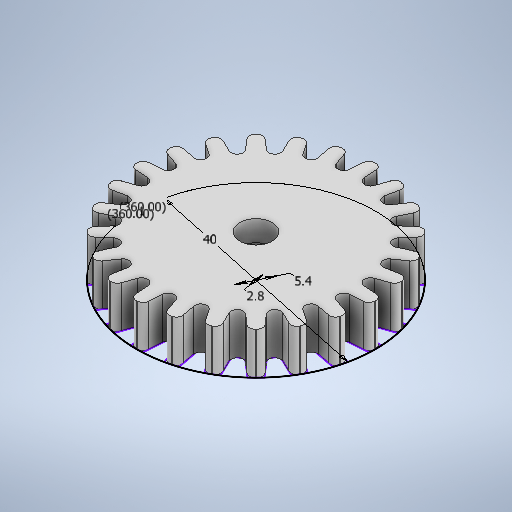
# Autodesk Inventor part: Direcccion3
Saved by Autodesk Inventor 2025.2 (Build 292293000, 293)
## iProperties
Created: 2025-03-19
Part Number: Direcccion3
Material: Genérico
Document SubType Name: Modeling
Designer: angel.dasilva
Density: 1 g/cm^3
Appearance: Valor por defecto
Author: angel.dasilva
Autodesk Inventor part; units mm, degrees
ref_plane "YZ Plane" through (0, 0, 0) normal (1, 0, 0) x (0, 1, 0)
ref_plane "XZ Plane" through (0, 0, 0) normal (0, 1, 0) x (-1, 0, 0)
ref_plane "XY Plane" through (0, 0, 0) normal (0, 0, 1) x (1, 0, 0)
sketch "Boceto1" plane through (0, 0, 0) normal (0, 1, 0) x (-1, 0, 0)
  circle A0 centre (0, 0) radius 20
  line L0 (20, 0) -> (19.975, -0.9997)
  line L1 (19.975, -0.9997) -> (15.9472, -1.2989)
  line L2 (20, 0) -> (19.975, 0.9997)
  line L3 (19.975, 0.9997) -> (15.9472, 1.2989)
  circle A1 centre (0, 0) radius 2.7
  circle A2 centre (0, 0) radius 1.4
  line L4 (19.0356, 6.1355) -> (15.0676, 5.3821)
  line L5 (19.5531, 4.2043) -> (15.74, 2.8728)
  line L6 (16.799, 10.8533) -> (13.1612, 9.0985)
  line L7 (17.7987, 9.1217) -> (14.4601, 6.8487)
  line L8 (13.4176, 14.8313) -> (10.3579, 12.1948)
  line L9 (14.8313, 13.4176) -> (12.1948, 10.3579)
  line L10 (9.1217, 17.7987) -> (6.8487, 14.4601)
  line L11 (10.8533, 16.799) -> (9.0985, 13.1612)
  line L12 (4.2043, 19.5531) -> (2.8728, 15.74)
  line L13 (6.1355, 19.0356) -> (5.3821, 15.0676)
  line L14 (-0.9997, 19.975) -> (-1.2989, 15.9472)
  line L15 (0.9997, 19.975) -> (1.2989, 15.9472)
  line L16 (-6.1355, 19.0356) -> (-5.3821, 15.0676)
  line L17 (-4.2043, 19.5531) -> (-2.8728, 15.74)
  line L18 (-10.8533, 16.799) -> (-9.0985, 13.1612)
  line L19 (-9.1217, 17.7987) -> (-6.8487, 14.4601)
  line L20 (-14.8313, 13.4176) -> (-12.1948, 10.3579)
  line L21 (-13.4176, 14.8313) -> (-10.3579, 12.1948)
  line L22 (-17.7987, 9.1217) -> (-14.4601, 6.8487)
  line L23 (-16.799, 10.8533) -> (-13.1612, 9.0985)
  line L24 (-19.5531, 4.2043) -> (-15.74, 2.8728)
  line L25 (-19.0356, 6.1355) -> (-15.0676, 5.3821)
  line L26 (-19.975, -0.9997) -> (-15.9472, -1.2989)
  line L27 (-19.975, 0.9997) -> (-15.9472, 1.2989)
  line L28 (-19.0356, -6.1355) -> (-15.0676, -5.3821)
  line L29 (-19.5531, -4.2043) -> (-15.74, -2.8728)
  line L30 (-16.799, -10.8533) -> (-13.1612, -9.0985)
  line L31 (-17.7987, -9.1217) -> (-14.4601, -6.8487)
  line L32 (-13.4176, -14.8313) -> (-10.3579, -12.1948)
  line L33 (-14.8313, -13.4176) -> (-12.1948, -10.3579)
  line L34 (-9.1217, -17.7987) -> (-6.8487, -14.4601)
  line L35 (-10.8533, -16.799) -> (-9.0985, -13.1612)
  line L36 (-4.2043, -19.5531) -> (-2.8728, -15.74)
  line L37 (-6.1355, -19.0356) -> (-5.3821, -15.0676)
  line L38 (0.9997, -19.975) -> (1.2989, -15.9472)
  line L39 (-0.9997, -19.975) -> (-1.2989, -15.9472)
  line L40 (6.1355, -19.0356) -> (5.3821, -15.0676)
  line L41 (4.2043, -19.5531) -> (2.8728, -15.74)
  line L42 (10.8533, -16.799) -> (9.0985, -13.1612)
  line L43 (9.1217, -17.7987) -> (6.8487, -14.4601)
  line L44 (14.8313, -13.4176) -> (12.1948, -10.3579)
  line L45 (13.4176, -14.8313) -> (10.3579, -12.1948)
  line L46 (17.7987, -9.1217) -> (14.4601, -6.8487)
  line L47 (16.799, -10.8533) -> (13.1612, -9.0985)
  line L48 (19.5531, -4.2043) -> (15.74, -2.8728)
  line L49 (19.0356, -6.1355) -> (15.0676, -5.3821)
  line L50 (19.975, -0.9997) -> (19.975, 0.9997)
  line L51 (19.5531, 4.2043) -> (19.0356, 6.1355)
  line L52 (17.7987, 9.1217) -> (16.799, 10.8533)
  line L53 (14.8313, 13.4176) -> (13.4176, 14.8313)
  line L54 (10.8533, 16.799) -> (9.1217, 17.7987)
  line L55 (6.1355, 19.0356) -> (4.2043, 19.5531)
  line L56 (0.9997, 19.975) -> (-0.9997, 19.975)
  line L57 (-4.2043, 19.5531) -> (-6.1355, 19.0356)
  line L58 (-9.1217, 17.7987) -> (-10.8533, 16.799)
  line L59 (-13.4176, 14.8313) -> (-14.8313, 13.4176)
  line L60 (-16.799, 10.8533) -> (-17.7987, 9.1217)
  line L61 (-19.0356, 6.1355) -> (-19.5531, 4.2043)
  line L62 (-19.975, 0.9997) -> (-19.975, -0.9997)
  line L63 (-19.5531, -4.2043) -> (-19.0356, -6.1355)
  line L64 (-17.7987, -9.1217) -> (-16.799, -10.8533)
  line L65 (-14.8313, -13.4176) -> (-13.4176, -14.8313)
  line L66 (-10.8533, -16.799) -> (-9.1217, -17.7987)
  line L67 (-6.1355, -19.0356) -> (-4.2043, -19.5531)
  line L68 (-0.9997, -19.975) -> (0.9997, -19.975)
  line L69 (4.2043, -19.5531) -> (6.1355, -19.0356)
  line L70 (9.1217, -17.7987) -> (10.8533, -16.799)
  line L71 (13.4176, -14.8313) -> (14.8313, -13.4176)
  line L72 (16.799, -10.8533) -> (17.7987, -9.1217)
  line L73 (19.0356, -6.1355) -> (19.5531, -4.2043)
  arc A3 (12.1948, -10.3579) -> (13.1612, -9.0985) centre (0, 0) ccw
  arc A4 (14.4601, -6.8487) -> (15.0676, -5.3821) centre (0, 0) ccw
  arc A5 (15.0676, 5.3821) -> (14.4601, 6.8487) centre (0, 0) ccw
  arc A6 (15.74, -2.8728) -> (15.9472, -1.2989) centre (0, 0) ccw
  arc A7 (15.9472, 1.2989) -> (15.74, 2.8728) centre (0, 0) ccw
  arc A8 (13.1612, 9.0985) -> (12.1948, 10.3579) centre (0, 0) ccw
  arc A9 (10.3579, 12.1948) -> (9.0985, 13.1612) centre (0, 0) ccw
  arc A10 (6.8487, 14.4601) -> (5.3821, 15.0676) centre (0, 0) ccw
  arc A11 (2.8728, 15.74) -> (1.2989, 15.9472) centre (0, 0) ccw
  arc A12 (-1.2989, 15.9472) -> (-2.8728, 15.74) centre (0, 0) ccw
  arc A13 (-5.3821, 15.0676) -> (-6.8487, 14.4601) centre (0, 0) ccw
  arc A14 (-9.0985, 13.1612) -> (-10.3579, 12.1948) centre (0, 0) ccw
  arc A15 (-12.1948, 10.3579) -> (-13.1612, 9.0985) centre (0, 0) ccw
  arc A16 (-14.4601, 6.8487) -> (-15.0676, 5.3821) centre (0, 0) ccw
  arc A17 (-15.74, 2.8728) -> (-15.9472, 1.2989) centre (0, 0) ccw
  arc A18 (-15.9472, -1.2989) -> (-15.74, -2.8728) centre (0, 0) ccw
  arc A19 (-15.0676, -5.3821) -> (-14.4601, -6.8487) centre (0, 0) ccw
  arc A20 (-13.1612, -9.0985) -> (-12.1948, -10.3579) centre (0, 0) ccw
  arc A21 (-10.3579, -12.1948) -> (-9.0985, -13.1612) centre (0, 0) ccw
  arc A22 (-6.8487, -14.4601) -> (-5.3821, -15.0676) centre (0, 0) ccw
  arc A23 (-2.8728, -15.74) -> (-1.2989, -15.9472) centre (0, 0) ccw
  arc A24 (1.2989, -15.9472) -> (2.8728, -15.74) centre (0, 0) ccw
  arc A25 (5.3821, -15.0676) -> (6.8487, -14.4601) centre (0, 0) ccw
  arc A26 (9.0985, -13.1612) -> (10.3579, -12.1948) centre (0, 0) ccw
  dimension "d0" = 40
  dimension "d4" = 1
  dimension "d10" = 5.4
  dimension "d54" = 2.8
  dimension "d62" = 360
  dimension "d66" = 360
  constraints: 148 end point, 50 point on circle, 27 centre point, 3 coincident, 1 vertical, 218 other
  measures "d0" diameter of A0
  measures "d4" distance of L0.start L0.end
  measures "d10" diameter of A1
  measures "d54" diameter of A2
extrude "Extrusión2" add sketch "Boceto1" along normal blind 3.5 contours A1
extrude "Extrusión4" add sketch "Boceto1" along normal blind 7 contours L50 L1 A6 L48 L73 L49 A4 L46 L72 L47 A3 L44 L71 L45 A26 L42 L70 L43 A25 L40 L69 L41 A24 L38 L68 L39 A23 L36 L67 L37 A22 L34 L66 L35 A21 L32 L65 L33 A20 L30 L64 L31 A19 L28 L63 L29 A18 L26 L62 L27 A17 L24 L61 L25 A16 L22 L60 L23 A15 L20 L59 L21 A14 L18 L58 L19 A13 L16 L57 L17 A12 L14 L56 L15 A11 L12 L55 L13 A10 L10 L54 L11 A9 L8 L53 L9 A8 L6 L52 L7 A5 L4 L51 L5 A7 L3
fillet "Empalme4" radius 1 30 edges at (-10.3579, 3.5, -12.1948) (-13.4176, 3.5, -14.8313) (-10.8533, 3.5, -16.799) (-9.1217, 3.5, -17.7987) (-6.8487, 3.5, -14.4601) (-5.3821, 3.5, -15.0676) (-6.1355, 3.5, -19.0356) (-9.0985, 3.5, -13.1612) (-14.8313, 3.5, -13.4176) (-17.7987, 3.5, -9.1217) (-16.799, 3.5, -10.8533) (-13.1612, 3.5, -9.0985) (-12.1948, 3.5, -10.3579) (-4.2043, 3.5, -19.5531) (-2.8728, 3.5, -15.74) (-1.2989, 3.5, -15.9472) (-0.9997, 3.5, -19.975) (0.9997, 3.5, -19.975) (2.8728, 3.5, -15.74) (4.2043, 3.5, -19.5531) (6.1355, 3.5, -19.0356) (9.1217, 3.5, -17.7987) (10.8533, 3.5, -16.799) (6.8487, 3.5, -14.4601) (5.3821, 3.5, -15.0676) (1.2989, 3.5, -15.9472) (10.3579, 3.5, -12.1948) (9.0985, 3.5, -13.1612) (13.4176, 3.5, -14.8313) (14.8313, 3.5, -13.4176)
fillet "Empalme5" radius 1 11 edges at (12.1948, 3.5, -10.3579) (13.1612, 3.5, -9.0985) (16.799, 3.5, -10.8533) (17.7987, 3.5, -9.1217) (14.4601, 3.5, -6.8487) (15.0676, 3.5, -5.3821) (19.0356, 3.5, -6.1355) (19.5531, 3.5, -4.2043) (15.74, 3.5, -2.8728) (15.9472, 3.5, -1.2989) (19.975, 3.5, -0.9997)
fillet "Empalme6" radius 1 8 edges at (19.975, 3.5, 0.9997) (15.74, 3.5, 2.8728) (19.5531, 3.5, 4.2043) (15.9472, 3.5, 1.2989) (19.0356, 3.5, 6.1355) (14.4601, 3.5, 6.8487) (15.0676, 3.5, 5.3821) (17.7987, 3.5, 9.1217)
fillet "Empalme7" radius 1 19 edges at (13.1612, 3.5, 9.0985) (12.1948, 3.5, 10.3579) (14.8313, 3.5, 13.4176) (16.799, 3.5, 10.8533) (13.4176, 3.5, 14.8313) (10.8533, 3.5, 16.799) (9.1217, 3.5, 17.7987) (9.0985, 3.5, 13.1612) (10.3579, 3.5, 12.1948) (6.8487, 3.5, 14.4601) (5.3821, 3.5, 15.0676) (6.1355, 3.5, 19.0356) (4.2043, 3.5, 19.5531) (-2.8728, 3.5, 15.74) (-1.2989, 3.5, 15.9472) (-0.9997, 3.5, 19.975) (0.9997, 3.5, 19.975) (1.2989, 3.5, 15.9472) (2.8728, 3.5, 15.74)
fillet "Empalme8" radius 1 28 edges at (-13.1612, 3.5, 9.0985) (-12.1948, 3.5, 10.3579) (-10.3579, 3.5, 12.1948) (-9.0985, 3.5, 13.1612) (-6.8487, 3.5, 14.4601) (-5.3821, 3.5, 15.0676) (-4.2043, 3.5, 19.5531) (-6.1355, 3.5, 19.0356) (-9.1217, 3.5, 17.7987) (-10.8533, 3.5, 16.799) (-13.4176, 3.5, 14.8313) (-14.8313, 3.5, 13.4176) (-16.799, 3.5, 10.8533) (-17.7987, 3.5, 9.1217) (-15.0676, 3.5, 5.3821) (-14.4601, 3.5, 6.8487) (-19.5531, 3.5, 4.2043) (-19.0356, 3.5, 6.1355) (-15.9472, 3.5, 1.2989) (-19.975, 3.5, 0.9997) (-19.975, 3.5, -0.9997) (-19.0356, 3.5, -6.1355) (-14.4601, 3.5, -6.8487) (-15.0676, 3.5, -5.3821) (-19.5531, 3.5, -4.2043) (-15.74, 3.5, -2.8728) (-15.9472, 3.5, -1.2989) (-15.74, 3.5, 2.8728)
